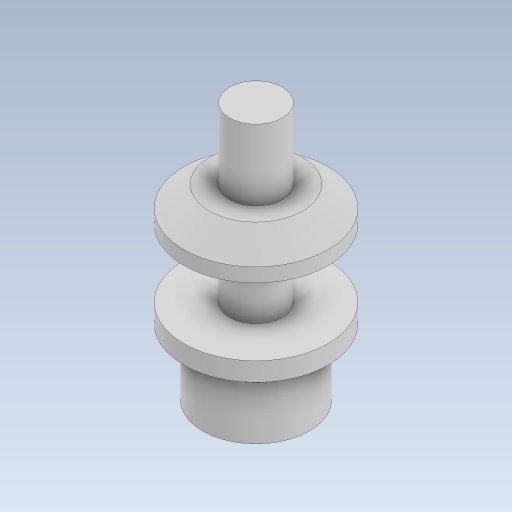
# Autodesk Inventor part: Drive Motor Shaft Coupler
Saved by Autodesk Inventor 2023 (Build 270158000, 158)
## iProperties
Created: 2023-01-21
Part Number: Drive Motor Shaft Coupler
Material: Generic
Document SubType Name: Modeling
Designer: Dave
Density: 1 g/cm^3
Appearance: Default
Author: Dave
Autodesk Inventor part; units mm, degrees
ref_plane "YZ Plane" through (0, 0, 0) normal (1, 0, 0) x (0, 1, 0)
ref_plane "XZ Plane" through (0, 0, 0) normal (0, 1, 0) x (-1, 0, 0)
ref_plane "XY Plane" through (0, 0, 0) normal (0, 0, 1) x (1, 0, 0)
sketch "Sketch1" plane through (0, 0, 0) normal (0, 0, 1) x (1, 0, 0)
  line L0 (3.75, 0) -> (7.25, 0)
  line L1 (7.25, 0) -> (7.25, 1.5)
  line L2 (7.25, 1.5) -> (10.05, 1.5)
  line L3 (10.05, 1.5) -> (10.05, 11.5)
  line L4 (10.05, 11.5) -> (13.55, 14)
  line L5 (13.55, 14) -> (13.55, 17.5)
  line L6 (13.55, 17.5) -> (5, 17.5)
  line L7 (5, 17.5) -> (5, 30.2)
  line L8 (5, 30.2) -> (13.55, 30.2)
  line L9 (13.55, 30.2) -> (13.55, 32.8)
  line L10 (13.55, 32.8) -> (8.75, 36.7)
  line L11 (8.75, 36.7) -> (5, 36.7)
  line L12 (5, 36.7) -> (5, 50)
  line L13 (5, 50) -> (0, 50)
  line L14 (0, 50) -> (0, 11.5)
  line L15 (3.75, 0) -> (3.75, 11.5)
  line L16 (3.75, 11.5) -> (0, 11.5)
  point P0 (0, 0)
  point P1 (2.5, 50)
  point P2 (1.875, 11.5)
  dimension "d0" = 3.75
  dimension "d1" = 3.5
  dimension "d2" = 1.5
  dimension "d3" = 2.8
  dimension "d4" = 10
  dimension "d5" = 3.5
  dimension "d6" = 2.5
  dimension "d7" = 3.5
  dimension "d8" = 5
  dimension "d9" = 12.7
  dimension "d10" = 2.6
  dimension "d11" = 3.9
  dimension "d12" = 4.8
  dimension "d13" = 50
  constraints: 34 end point, 9 perpendicular, 4 point on line, 2 horizontal alignment, 2 midpoint, 2 parallel, 2 vertical alignment, 1 horizontal, 1 vertical
  measures "d0" distance of point (0, 0) L0.start
  measures "d1" distance of L0.start L0.end
  measures "d2" distance of L0.end L1.end
  measures "d3" distance of L1.end L2.end
  measures "d4" distance of L2.end L3.end
  measures "d5" horizontal distance of L4.end L3.end
  measures "d6" vertical distance of L4.end L3.end
  measures "d7" distance of L4.end L5.end
  measures "d8" distance from line of point (0, 0) L7
  measures "d9" distance of L6.end L7.end
  measures "d10" distance of L8.end L9.end
  measures "d11" vertical distance of L10.end L9.end
  measures "d12" horizontal distance of L10.end L9.end
  measures "d13" vertical distance of point (0, 0) point (2.5, 50)
revolve "Revolution1" add sketch "Sketch1" angle 360 about axis through (0, 50, 0) along (0, -1, 0)
body "Solid1"
